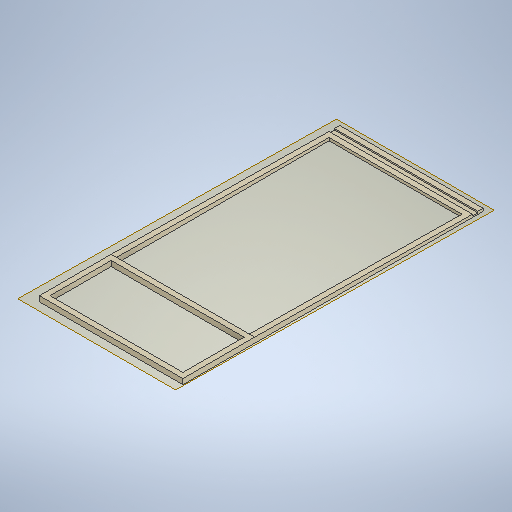
# Autodesk Inventor part: wing1.1
Saved by Autodesk Inventor 2025 (Build 290162000, 162)
## iProperties
Created: 2026-07-27
Part Number: wing1.1
Material: Generic
Document SubType Name: Modeling
Designer: DSTJOHN
Density: 1 g/cm^3
Appearance: Default
Author: DSTJOHN
Autodesk Inventor part; units mm, degrees
ref_plane "YZ Plane" through (0, 0, 0) normal (1, 0, 0) x (0, 1, 0)
ref_plane "XZ Plane" through (0, 0, 0) normal (0, 1, 0) x (-1, 0, 0)
ref_plane "XY Plane" through (0, 0, 0) normal (0, 0, 1) x (1, 0, 0)
sketch "Sketch1" plane through (0, 0, 0) normal (0, 1, 0) x (-1, 0, 0)
  line L0 (0, 0) -> (-50, 0)
  line L1 (-50, 0) -> (-50, -105)
  line L2 (-50, -105) -> (0, -105)
  line L3 (0, -105) -> (0, 0)
  line L4 (2, 2) -> (-52, 2)
  line L5 (-52, 2) -> (-52, -104)
  line L6 (2, -104) -> (2, 2)
  line L7 (2, -104) -> (2, -111)
  line L8 (2, -111) -> (-52, -111)
  line L9 (-52, -111) -> (-52, -102)
  dimension "d0" = 50
  dimension "d1" = 105
  dimension "d23" = 6
  dimension "d24" = 2
  constraints: 20 end point, 3 parallel, 3 perpendicular, 2 horizontal, 1 point on line, 1 vertical
  measures "d0" distance between parallel lines of L1 L3
  measures "d1" distance between parallel lines of L2 L0
  measures "d23" distance between parallel lines of L8 L2
  measures "d24" distance between parallel lines of L4 L0
extrude "Extrusion1" add sketch "Sketch1" along normal blind 2
ref_plane "Work Plane1" through (45, 2, -25) normal (0, 0.9999, -0.0117) x (-1, 0, 0)
sketch "Sketch3" plane through (45, 2, -25) normal (0, 0.9999, -0.0117) x (-1, 0, 0)
  line L0 (51, 33) -> (-14, 33)
  line L1 (-14, 33) -> (-14, -92)
  line L2 (-14, -92) -> (51, -92)
  line L3 (51, -92) -> (51, 33)
  point P0 (45, 24.9749)
  constraints: 8 end point, 2 parallel, 1 horizontal, 1 perpendicular
extrude "Extrusion3" cut sketch "Sketch3" along normal blind 2
sketch "Sketch7" plane through (45, 2, -25) normal (0, 0.9999, -0.0117) x (-1, 0, 0)
  line L0 (47, -86.0175) -> (47, 26.9748) projected
  line L1 (47, -82) -> (-7, -82)
  line L2 (-7, -82) -> (-7, -84)
  line L3 (-7, -84) -> (47, -84)
  line L4 (47, -84) -> (47, -82)
  point P0 (45, 24.9749)
  constraints: 8 end point, 2 parallel, 1 horizontal, 1 perpendicular, 1 point on line
extrude "Extrusion6" cut sketch "Sketch7" against normal blind 0.5
sketch "Sketch8" plane through (0, 0, 0) normal (0, -1, 0) x (1, 0, 0)
  line L0 (50, -25) -> (50, 0) construction
  line L1 (50, 0) -> (50, -105) construction
  line L2 (50, -105) -> (50, -25) construction
  line L3 (50, -25) -> (50, -105) projected
  line L4 (50, -25) -> (0, -25)
  line L5 (0, -25) -> (0, -23)
  line L6 (0, -23) -> (50, -23)
  line L7 (50, -23) -> (50, -25)
  point P0 (0, 0)
  constraints: 12 end point, 2 parallel, 1 horizontal, 1 perpendicular
extrude "Extrusion7" add sketch "Sketch8" against normal blind 2
body "Solid1"
